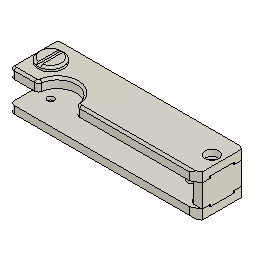
Summit (Autodesk Fusion 360 design; units mm, degrees)
Autodesk Fusion 360 part; units mm, degrees
sketch "Faceplate_Profile" plane through (0, 0, 0) normal (0, 0, 1) x (1, 0, 0)
  line L0 (0, 0) -> (90, 0)
  line L1 (90, 0) -> (90, 23)
  line L2 (90, 23) -> (0, 23)
  line L3 (0, 23) -> (0, 0)
  arc A0 (31.5, 0) -> (13.5, 0) centre (22.5, 0.1978) ccw
  line L4 (22.5, 0.1978) -> (22.5, 9.2) construction
  circle A1 centre (93, 11.5) radius 12 construction
  line L5 (90, 11.5) -> (93, 11.5) construction
  line L6 (85.7138, 21.0347) -> (85.7138, 1.9653)
  line L7 (85.7138, 1.9653) -> (91.3268, -2.3241) construction
  line L8 (85.7138, 21.0347) -> (90.4142, 24.6266) construction
  arc A2 (85.7138, 21.0347) -> (85.7138, 1.9653) centre (93, 11.5) ccw
  line L9 (89.2138, 26.5305) -> (89.2138, -3.5305) construction
  arc A3 (89.2138, 26.5305) -> (89.2138, -3.5305) centre (93, 11.5) ccw construction
  line L10 (77.5, 23) -> (77.5, 0) construction
  line L11 (85.7138, 1.9653) -> (77.5, 1.9653)
  line L12 (77.5, 1.9653) -> (77.5, 21.0347)
  line L13 (77.5, 21.0347) -> (85.7138, 21.0347)
  line L14 (85.7138, 21.0347) -> (85.7138, 1.9653)
  circle A4 centre (75.5, 11.5) radius 2
  line L15 (85.7138, 21.0347) -> (90, 21.0347)
  line L16 (85.7138, 1.9653) -> (85, 1.9653)
  circle A5 centre (8, 11.5) radius 6
  line L17 (0, 11.5) -> (8, 11.5) construction
  line L18 (7, 17.4161) -> (7, 5.5839)
  line L19 (9, 17.4161) -> (9, 5.5839)
  line L20 (9, 11.5) -> (7, 11.5) construction
  circle A6 centre (8, 11.5) radius 3.8
  line L21 (75.5, 11.5) -> (77.5, 11.5) construction
  line L22 (85.7138, 1.9653) -> (90, 1.9653)
  dimension "d12" = 90
  dimension "d13" = 23
  dimension "d14" = 9.2
  dimension "d16" = 22.5
  dimension "d17" = 18
  dimension "d42" = 24
  dimension "d43" = 3
  dimension "d45" = 4
  dimension "d106" = 12
  dimension "d107" = 7.6
  dimension "d121" = 7.2862
  dimension "d122" = 3.5
  dimension "d123" = 8
  dimension "d124" = 2
  constraint horizontal L0
  constraint vertical L1
  constraint horizontal L2
  constraint vertical L3
  constraint coincident L0.start L3.end
  constraint coincident L0 A0.end
  constraint coincident L0 A0.start
  constraint coincident A0.centre L4.start
  constraint midpoint A0 L4.end
  constraint midpoint L1 L5.start
  constraint coincident A1.centre L5.end
  constraint horizontal L5
  constraint coincident A1 L6.start
  constraint coincident A1 L6.end
  constraint vertical L6
  constraint tangent A1 L8
  constraint tangent A1 L7
  constraint tangent L7 A2
  constraint coincident L2 L10.start
  constraint coincident L0 L10.end
  constraint perpendicular L0 L10
  constraint horizontal L11
  constraint vertical L12
  constraint horizontal L13
  constraint vertical L14
  constraint tangent L12 A4
  constraint coincident L1 L15.end
  constraint perpendicular L1 L15
  constraint perpendicular L6 L16
  constraint midpoint L3 L17.start
  constraint coincident A5.centre L17.end
  constraint horizontal L17
  constraint coincident A5 L18.start
  constraint coincident A5 L18.end
  constraint vertical L18
  constraint coincident A5 L19.start
  constraint coincident A5 L19.end
  constraint parallel L18 L19
  constraint midpoint L19 L20.start
  constraint midpoint L18 L20.end
  constraint midpoint A5.centre L20
  constraint concentric A5 A6
  constraint concentric A2 A3
  constraint tangent A3 L10
  constraint collinear L10 L12
  constraint collinear L13 L15
  constraint coincident A4.centre L21.start
  constraint coincident L12 L21.end
  constraint horizontal L21
  constraint midpoint L10 L21.end
  constraint coincident L1 L22.end
  constraint perpendicular L1 L22
  measures "d12" distance of L0.start L0.end
  measures "d13" distance of L0.start L2.end
  measures "d14" distance of L0 L4.end
  measures "d16" horizontal distance of L0.start A0.centre
  measures "d17" distance of A0.end A0.start
  measures "d42" diameter of A1
  measures "d43" distance of L1 A1.centre
  measures "d45" diameter of A4
  measures "d106" diameter of A5
  measures "d107" diameter of A6
  measures "d121" distance of L6 A1.centre
  measures "d122" distance of A1 A3
  measures "d123" distance of L3 A5.centre
  measures "d124" distance of L18 L19
extrude "Extrude1" add sketch "Faceplate_Profile" along normal blind 4.6 contours A4 | L0 L1 L2 L3 A0 L11 L12 L13 L15 L16 L22 | L1 L6 L14 L15 L22 | L6 A2 L14 | A2 L11 L12 L13 L16 | A5 L19 A6 | A5 L18 L19 A6 | A5 L18 L19 A6 | A5 L18 A6 | L19 A6 | L18 L19 A6 | L18 A6 makes body 1 in component "Plate_Top"
extrude "Extrude1'" add sketch "Faceplate_Profile" against normal blind 4.6 from surface at -10.8 separate body contours A4 | L0 L1 L2 L3 A0 L11 L12 L13 L15 L16 L22 | L0 A0 | L1 L6 L14 L15 L22 | L6 A2 L14 | A2 L11 L12 L13 L16 | A5 L19 A6 | A5 L18 L19 A6 | A5 L18 L19 A6 | A5 L18 A6 | L19 A6 | L18 L19 A6 | L18 A6 makes body 2 in component "Plate_Bottom"
extrude "Extrude1''" add sketch "Faceplate_Profile" against normal up to surface (10.8 mm away) separate body contours A4 | L1 L6 L14 L15 L22 | L6 A2 L14 makes body 3 at (85.273, 2.3188, -7.2) makes body 4 at (73.9057, 10.2924, -7.2) in component "Ring_Holder"
sketch "Holder things" plane through (0, 0, -10.8) normal (0, 0, 1) x (-1, 0, 0) in component "Ring_Holder"
  line L0 (-90, 0) -> (-90, -23)
  line L1 (-90, -23) -> (0, -23)
  line L2 (0, -23) -> (0, 0)
  line L3 (0, 0) -> (-90, 0)
  arc A0 (-85.7138, -21.0347) -> (-85.7138, -1.9653) centre (-93, -11.5) ccw
  line L4 (-90, -1.9653) -> (-90, -21.0347)
  line L5 (0, 0) -> (-90, 0)
  line L6 (-90, 0) -> (-90, -23)
  line L7 (0, -23) -> (0, 0)
  line L8 (-90, -23) -> (0, -23)
  line L9 (-82.4, -17.1249) -> (-82.4, -5.8751)
  line L10 (-82.4, -5.8751) -> (-90, -5.8751)
  line L11 (-90, -5.8751) -> (-90, -17.1249)
  line L12 (-90, -17.1249) -> (-82.4, -17.1249)
  circle A1 centre (-85.2, -11.5) radius 1.5
  line L13 (-82.4, -11.5) -> (-90, -11.5) construction
  circle A2 centre (-75.5, -11.5) radius 1.5
  line L14 (-85.7138, -1.9653) -> (-90, -1.9653)
  line L15 (-90, -21.0347) -> (-85.7138, -21.0347)
  circle A3 centre (-75.5, -11.5) radius 2
  point P0 (-75.5, -11.5)
  dimension "d49" = 3
  dimension "d126" = 4.8
  dimension "d128" = 3
  dimension "d130" = 2.8
  constraint perpendicular L9 L10
  constraint parallel L9 L11
  constraint parallel L10 L12
  constraint coincident A0 L9.end
  constraint vertical L9
  constraint coincident A0 L9.start
  constraint midpoint L9 L13.start
  constraint midpoint L4 L13.end
  constraint coincident A1.centre L13
  constraint collinear L0 L11
  constraint coincident P0 A2.centre
  measures "d49" diameter of A1
  measures "d126" distance of L11 A1.centre
  measures "d128" diameter of A2
  measures "d130" distance of L9 A1.centre
extrude "Extrude2" cut sketch "Holder things" along normal blind -1 and the other way blind 0 contours L0 L4 L6 L9 L10 L11 L12 | A1 bodies 2 in component "Plate_Bottom"
extrude "Extrude2'" cut sketch "Holder things" along normal blind 1 from surface at 10.8 contours L0 L4 L6 L9 L10 L11 L12 | A1 bodies 1 in component "Plate_Top"
extrude "Extrude2''" add sketch "Holder things" against normal blind 1 contours L0 L4 L6 L9 L10 L11 L12 bodies 3 in component "Ring_Holder"
extrude "Extrude3" add sketch "Holder things" along normal blind 1 from surface at 10.8 contours L0 L4 L6 L9 L10 L11 L12 bodies 3 in component "Ring_Holder"
move_face "OffsetFaces1" offset -0.2 3 faces at (87.4667, 17.1249, -11.1333) (84.9333, 5.8751, -11.1333) (82.4, 13.375, -11.4667) on bodies 2 in component "Plate_Bottom"
move_face "OffsetFaces1'" offset -0.2 3 faces at (82.4, 13.375, 0.3333) (84.9333, 17.1249, 0.6667) (87.4667, 5.8751, 0.6667) on bodies 1 in component "Plate_Top"
sketch "D_plate_bores" plane through (0, 0, 4.6) normal (0, 0, 1) x (-1, 0, 0) in component "Ring_Holder"
  line L0 (-90, 0) -> (-90, -23)
  line L1 (-90, -23) -> (0, -23)
  line L2 (0, -23) -> (0, 0)
  line L3 (0, 0) -> (-13.5, 0)
  arc A0 (-31.5, 0) -> (-13.5, 0) centre (-22.5, -0.1978) ccw
  line L4 (-31.5, 0) -> (-90, 0)
  circle A1 centre (-75.5, -11.5) radius 2
  circle A2 centre (-75.5, -11.5) radius 2
  line L5 (-90, -5.8751) -> (-90, -17.1249)
  line L6 (-90, -17.1249) -> (-82.4, -17.1249)
  line L7 (-82.4, -17.1249) -> (-82.4, -5.8751)
  line L8 (-82.4, -5.8751) -> (-90, -5.8751)
  circle A3 centre (-85.2, -11.5) radius 1.5
hole "Hole1" at (85.2, 11.5, 4.6) direction (0, 0, -1) diameter 3.4 depth 19 tip angle 180 counterbore diameter 6.5 counterbore depth 3 bodies 1 in component "Plate_Top"
hole "Hole1'" at (85.2, 11.5, 4.6) direction (0, 0, -1) diameter 3.4 depth 19 tip angle 180 counterbore diameter 6.5 counterbore depth 3 bodies 2 in component "Plate_Bottom"
hole "Hole1''" at (85.2, 11.5, 4.6) direction (0, 0, -1) diameter 3.4 depth 19 tip angle 180 counterbore diameter 6.5 counterbore depth 3 bodies 3 in component "Ring_Holder"
sketch "D_plate_nut" plane through (0, 0, -15.4) normal (0, 0, 1) x (-1, 0, 0) in component "Plate_Bottom"
  line L0 (0, 0) -> (0, -23)
  line L1 (0, -23) -> (-90, -23)
  line L2 (-90, -23) -> (-90, 0)
  line L3 (-90, 0) -> (0, 0)
  circle A0 centre (-85.2, -11.5) radius 1.7
  line L4 (-88.1, -13.1743) -> (-85.2, -14.8486)
  line L5 (-85.2, -14.8486) -> (-82.3, -13.1743)
  line L6 (-82.3, -13.1743) -> (-82.3, -9.8257)
  line L7 (-82.3, -9.8257) -> (-85.2, -8.1514)
  line L8 (-85.2, -8.1514) -> (-88.1, -9.8257)
  line L9 (-88.1, -9.8257) -> (-88.1, -13.1743)
  circle A1 centre (-75.5, -11.5) radius 1.5
  circle A2 centre (-75.5, -11.5) radius 2
  point P0 (-83.5894, -10.9561)
  point P1 (-85.2, -11.5)
  dimension "d101" = 2.9
  dimension "d129" = 4
  constraint coincident P0 A0
  constraint coincident P1 A0.centre
  constraint vertical L9
  constraint concentric A1 A2
  measures "d101" distance of P1 L9
  measures "d129" diameter of A2
extrude "Extrude3'" cut sketch "D_plate_nut" along normal blind 2.8 from surface at 0.4 contours A0 | L4 L5 L6 L7 L8 L9 bodies 2 in component "Plate_Bottom"
hole "Hole2" at (75.5, 11.5, -15.4) direction (0, 0, 1) diameter 3.2 depth 19.2 tip angle 180 counterbore diameter 6.5 counterbore depth 3 bodies 1 in component "Plate_Top"
hole "Hole2'" at (75.5, 11.5, -15.4) direction (0, 0, 1) diameter 3.2 depth 19.2 tip angle 180 counterbore diameter 6.5 counterbore depth 3 bodies 2 in component "Plate_Bottom"
hole "Hole2''" at (75.5, 11.5, -15.4) direction (0, 0, 1) diameter 3.2 depth 19.2 tip angle 180 counterbore diameter 6.5 counterbore depth 3 bodies 4 in component "Ring_Holder"
sketch "Key_standoff" plane through (0, 0, 4.6) normal (0, 0, 1) x (-1, 0, 0) in component "Plate_Top"
  line L0 (-90, 0) -> (-90, -23)
  line L1 (-90, -23) -> (0, -23)
  line L2 (0, -23) -> (0, 0)
  line L3 (0, 0) -> (-13.5, 0)
  arc A0 (-31.5, 0) -> (-13.5, 0) centre (-22.5, -0.1978) ccw
  line L4 (-31.5, 0) -> (-90, 0)
  circle A1 centre (-8, -11.5) radius 6
  circle A2 centre (-8, -11.5) radius 3.8
  line L5 (-9, -17.4161) -> (-9, -5.5839)
  line L6 (-7, -17.4161) -> (-7, -5.5839)
  circle A3 centre (-85.2, -11.5) radius 3.25
extrude "Extrude4" cut sketch "Key_standoff" against normal blind 3 contours A1 A2 L6 | A1 A2 L5 L6 | A1 A2 L5 L6 | A1 A2 L5 bodies 1 in component "Plate_Top"
hole "Hole3" at (8, 11.5, 4.6) direction (0, 0, -1) diameter 3.2 end through all counterbore diameter 6.5 counterbore depth 3 bodies 2 1 in component "Plate_Top"
hole "Hole3'" at (8, 11.5, 4.6) direction (0, 0, -1) diameter 3.2 end through all counterbore diameter 6.5 counterbore depth 3 bodies 2 in component "Plate_Bottom"
extrude "Extrude1'''" add sketch "Key_standoff" along normal blind 2 separate body contours A1 A2 L6 | A1 A2 L5 L6 | A1 A2 L5 L6 | A1 A2 L5 | A2 L5 L6 | A2 L6 | A2 L5 makes body 5 in component "Keyhole_Cap"
chamfer "Chamfer2" distance 1 angle 45 1 edges at (13.594, 13.6697, 6.6) on bodies 5 in component "Keyhole_Cap"
extrude "Extrude2'''" cut sketch "Key_standoff" along normal blind 2 from surface at 1 contours A1 A2 L5 L6 | A1 A2 L5 L6 | A2 L5 L6 bodies 5 in component "Keyhole_Cap"
extrude "Extrude3''" add sketch "Key_standoff" against normal up to surface (2.4 mm away) contours A1 A2 L6 | A1 A2 L5 L6 | A1 A2 L5 L6 | A1 A2 L5 bodies 5 in component "Keyhole_Cap"
sketch "Key_standoff_nut" plane through (0, 0, -15.4) normal (0, 0, -1) x (1, 0, 0) in component "Plate_Bottom"
  circle A0 centre (8, -11.5) radius 1.6
  line L0 (0, 0) -> (0, -23)
  line L1 (0, -23) -> (90, -23)
  line L2 (90, -23) -> (90, 0)
  line L3 (90, 0) -> (0, 0)
  circle A1 centre (8, -11.5) radius 6
  circle A2 centre (8, -11.5) radius 3.8
  line L4 (9, -17.4161) -> (9, -5.5839)
  line L5 (7, -17.4161) -> (7, -5.5839)
  line L6 (9.6743, -8.6) -> (6.3257, -8.6)
  line L7 (6.3257, -8.6) -> (4.6514, -11.5)
  line L8 (4.6514, -11.5) -> (6.3257, -14.4)
  line L9 (6.3257, -14.4) -> (9.6743, -14.4)
  line L10 (9.6743, -14.4) -> (11.3486, -11.5)
  line L11 (11.3486, -11.5) -> (9.6743, -8.6)
  circle A3 centre (75.5, -11.5) radius 3.25
  point P0 (8, -11.5)
  dimension "d118" = 2.9
  constraint coincident P0 A0.centre
  constraint horizontal L9
  measures "d118" distance of P0 L11
extrude "Extrude4'" cut sketch "Key_standoff_nut" against normal blind 3 contours A0 L4 L6 L9 L10 L11 | A0 L4 L5 L6 | A0 L4 L5 L9 | A0 L5 L6 L7 L8 L9 | A1 A2 L4 | A1 A2 L4 L5 | A1 A2 L4 L5 | A1 A2 L5 bodies 2 in component "Plate_Bottom"
sketch "Midpost_nut" plane through (0, 0, 0) normal (0, 0, -1) x (1, 0, 0) in component "Plate_Top"
  line L0 (82.2, -5.6751) -> (90, -5.6751)
  line L1 (90, -5.6751) -> (90, 0)
  line L2 (90, 0) -> (31.5, 0)
  arc A0 (13.5, 0) -> (31.5, 0) centre (22.5, -0.1978) ccw
  line L3 (13.5, 0) -> (0, 0)
  line L4 (0, 0) -> (0, -23)
  line L5 (0, -23) -> (90, -23)
  line L6 (90, -23) -> (90, -17.3249)
  line L7 (90, -17.3249) -> (82.2, -17.3249)
  line L8 (82.2, -17.3249) -> (82.2, -5.6751)
  line L9 (77.1743, -8.6) -> (73.8257, -8.6)
  line L10 (73.8257, -8.6) -> (72.1514, -11.5)
  line L11 (72.1514, -11.5) -> (73.8257, -14.4)
  line L12 (73.8257, -14.4) -> (77.1743, -14.4)
  line L13 (77.1743, -14.4) -> (78.8486, -11.5)
  line L14 (78.8486, -11.5) -> (77.1743, -8.6)
  circle A1 centre (8, -11.5) radius 1.6
  circle A2 centre (75.5, -11.5) radius 1.6
  circle A3 centre (75.5, -11.5) radius 1.6
  point P0 (75.5, -11.5)
  dimension "d102" = 2.9
  constraint coincident P0 A2.centre
  constraint horizontal L12
  measures "d102" distance of P0 L14
extrude "Extrude3'''" cut sketch "Midpost_nut" against normal blind 2.8 from surface at -1 contours L9 L10 L11 L12 L13 L14 bodies 1 in component "Plate_Top"
fillet "Fillet1" radius 2 2 edges at (0, 23, -13.1) (0, 0, -13.1) on bodies 2 in component "Plate_Bottom"
fillet "Fillet1'" radius 2 4 edges at (13.5, 0, 2.3) (31.5, 0, 2.3) (0, 0, 2.3) (0, 23, 2.3) on bodies 1 in component "Plate_Top"
chamfer "Chamfer1" distance 4 distance2 2 1 edges at (90, 23, -13.1) measured on face at (31.3333, 23, -13.8667) on bodies 2 in component "Plate_Bottom"
chamfer "Chamfer1" distance 2 distance2 4 1 edges at (90, 0, -13.1) measured on face at (90, 9.5584, -14.2) on bodies 2 in component "Plate_Bottom"
chamfer "Chamfer1" distance 1 distance2 1 5 edges at (46, 0, -15.4) (0.5858, 0.5858, -15.4) (0, 11.5, -15.4) (0.5858, 22.4142, -15.4) (46, 23, -15.4) measured on face at (86.247, 11.419, -15.4) measured on face at (1.9048, 0.0023, -13.8667) measured on face at (86.247, 11.419, -15.4) measured on face at (0.0023, 21.0952, -13.8667) measured on face at (86.247, 11.419, -15.4) on bodies 2 in component "Plate_Bottom"
chamfer "Chamfer1'" distance 4 distance2 2 1 edges at (90, 0, 2.3) measured on face at (52.2357, 0, 1.5333) on bodies 1 in component "Plate_Top"
chamfer "Chamfer1'" distance 2 distance2 4 1 edges at (90, 23, 2.3) measured on face at (90, 9.5584, 3.4) on bodies 1 in component "Plate_Top"
chamfer "Chamfer1'" distance 1 distance2 1 9 edges at (6.8232, 0, 4.6) (12.9396, 0.4744, 4.6) (22.5, 9.2, 4.6) (32.0604, 0.4744, 4.6) (61.6768, 0, 4.6) (46, 23, 4.6) (0.5858, 22.4142, 4.6) (0, 11.5, 4.6) (0.5858, 0.5858, 4.6) measured on face at (68.781, 3.0392, 4.6) measured on face at (12.291, 0.1067, 1.5333) measured on face at (68.781, 3.0392, 4.6) measured on face at (32.8891, 0.0547, 1.5333) measured on face at (68.781, 3.0392, 4.6) measured on face at (68.781, 3.0392, 4.6) measured on face at (0.0023, 21.0952, 1.5333) measured on face at (68.781, 3.0392, 4.6) measured on face at (1.9048, 0.0023, 1.5333) on bodies 1 in component "Plate_Top"
component "Plate_Top" placed x (1, 0, 0) y (0, 1, 0) z (0, 0, 1) at (0, 0, 0)
component "Plate_Bottom" placed x (1, 0, 0) y (0, 1, 0) z (0, 0, 1) at (0, 0, 0)
component "Ring_Holder" placed x (1, 0, 0) y (0, 1, 0) z (0, 0, 1) at (0, 0, 0)
component "Keyhole_Cap" placed x (1, 0, 0) y (0, 1, 0) z (0, 0, 1) at (0, 0, 0) in component "Plate_Top"
equation "Key_Length = 70 mm" comment "Max length of key"
equation "Key_Width = 28 mm" comment "Max width of key"
equation "Key_Thicc = 2,8 mm" comment "Max thickness of key"
equation "Case_Width = Key_Width - 5 mm" comment "Full width of case"
equation "Case_Length = Key_Length + 20 mm" comment "Full length of case"
equation "Plate_Thicc = 4,6 mm" comment "Thickness of each case plate"
equation "Plate_Spacing = ( ( Key_Thicc + 0,6 mm ) * Key_Count ) + 0,6 mm" comment "Full extent of space that will accomodate the keys"
equation "Key_Count = 3" comment "Number of keys to fit inside keyring"
equation "Finger_indent = Case_Width * 2 / 5"
equation "Ring_ID = 24 mm" comment "Inner Diameter of keychain ring"
equation "Ring_Thickness = 3 mm"
equation "d12 = Case_Length"
equation "d13 = Case_Width"
equation "d14 = Finger_indent"
equation "d16 = ( Case_Length / 4 mm ) * 1 mm"
equation "d18 = Plate_Thicc"
equation "d23 = -Plate_Spacing"
equation "d24 = -Plate_Thicc"
equation "d42 = Ring_ID"
equation "d43 = Ring_ID / 8"
equation "d51 = -Plate_Thicc + 3,6 mm"
equation "d56 = -d51"
equation "d58 = d51"
equation "d61 = -d51"
equation "d77 = 2 * Plate_Thicc + Plate_Spacing - 1 mm"
equation "d78 = 2 * Plate_Thicc + Plate_Spacing - 1 mm"
equation "d79 = 2 * Plate_Thicc + Plate_Spacing - 1 mm"
equation "d84 = 2,8 mm"
equation "d86 = 2 * Plate_Thicc + Plate_Spacing - 0,8 mm"
equation "d91 = 2 * Plate_Thicc + Plate_Spacing - 0,8 mm"
equation "d96 = 2 * Plate_Thicc + Plate_Spacing - 0,8 mm"
equation "d101 = ( 5,8 / 2 ) * 1 mm"
equation "d102 = ( 5,8 / 2 ) * 1 mm"
equation "d104 = -d84"
equation "d108 = -Plate_Thicc + 1,6 mm"
equation "d118 = ( 5,8 / 2 ) * 1 mm"
